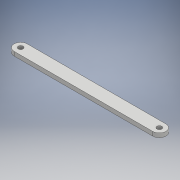
# Autodesk Inventor part: passiveLink
Saved by Autodesk Inventor 2018 (Build 220112000, 112)
## iProperties
Created: 2017-12-31
Part Number: passiveLink
Material: Generic
Document SubType Name: Modeling
Designer: mzhang
Density: 1 g/cm^3
Appearance: Default
Author: mzhang
Autodesk Inventor part; units mm, degrees
ref_plane "YZ Plane" through (0, 0, 0) normal (1, 0, 0) x (0, 1, 0)
ref_plane "XZ Plane" through (0, 0, 0) normal (0, 1, 0) x (-1, 0, 0)
ref_plane "XY Plane" through (0, 0, 0) normal (0, 0, 1) x (1, 0, 0)
sketch "Sketch1" plane through (0, 0, 0) normal (0, 0, 1) x (1, 0, 0)
  circle A0 centre (0, 0) radius 1.778
  circle A1 centre (101.6, 0) radius 1.778
  line L0 (4.2559, 2.1718) -> (97.3441, 2.1718)
  line L1 (101.6, 3.222) -> (101.6, -1.778)
  line L2 (97.5368, -2.5139) -> (4.0632, -2.5139)
  line L3 (0, -3.222) -> (0, 1.778)
  arc A2 (4.2559, 2.1718) -> (4.0632, -2.5139) centre (0, 0) ccw
  arc A3 (97.5368, -2.5139) -> (97.3441, 2.1718) centre (101.6, 0) ccw
  line L4 (0, 4.778) -> (101.6, 4.778)
  line L5 (101.6, -4.778) -> (0, -4.778)
  dimension "d0" = 3.556
  dimension "d1" = 3.556
  dimension "d2" = 101.6
  dimension "d3" = 3
  dimension "d4" = 3
  constraints: 12 end point, 8 point on circle, 3 parallel, 2 centre point, 2 horizontal, 2 tangent, 2 vertical alignment, 1 coincident, 1 perpendicular, 4 other
  measures "d2" distance of A3.centre point (0, 0)
extrude "Extrusion1" add sketch "Sketch1" along normal blind 3
body "Solid1"
